Autodesk Inventor part; units mm, degrees
(part 2 of 2)
extrude "拉伸43" cut sketch "position草图" against normal through all contours L5 L7 L6 L8 bodies 7
extrude "拉伸44" cut sketch "position草图" against normal through all contours L33 L36 L35 L11 L10 | L10 L11 L35 L34 L33 | L39 L42 L41 L12 L11 | L11 L12 L41 L40 L39 | L14 L52 L51 L13 | L13 L51 L54 L53 L14 | L75 L78 L77 L16 L15 | L15 L16 L77 L76 | L105 L108 L107 L17 L16 | L16 L17 L107 L106 L105 | L87 L90 L89 L19 L18 | L18 L19 L89 L88 | L93 L96 L95 L20 L19 | L19 L20 L95 L94 L93 | L24 L23 L22 L21 | L30 L29 L28 L27 | L48 L47 L46 L45 | L60 L59 L58 L57 | L66 L65 L64 L63 | L72 L71 L70 L69 | L84 L83 L82 L81 | L102 L101 L100 L99 | L114 L113 L112 L111 | L120 L119 L118 L117 | L126 L125 L124 L123 | L132 L131 L130 L129 bodies 7
